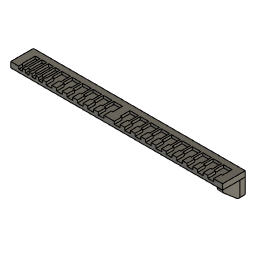
CClampRack v7 (Autodesk Fusion 360 design; units mm, degrees)
Autodesk Fusion 360 part; units mm, degrees
sketch "Sketch1" plane through (0, 0, 0) normal (0, 0, 1) x (1, 0, 0)
  line L0 (0, 76.2) -> (0, 0)
  line L1 (114.3, 57.15) -> (142.875, 57.15)
  line L2 (142.875, 57.15) -> (142.875, 25.4)
  line L3 (142.875, 25.4) -> (114.3, 25.4)
  line L4 (114.3, 25.4) -> (114.3, 57.15)
  line L5 (128.5875, 25.4) -> (128.5875, 0) construction
  line L6 (119.0625, 25.4) -> (119.0625, 0)
  line L7 (138.1125, 25.4) -> (138.1125, 0)
  line L8 (25.4, 57.15) -> (25.4, 12.7)
  line L9 (25.4, 12.7) -> (41.275, 12.7)
  line L10 (41.275, 12.7) -> (41.275, 57.15)
  line L11 (26.9875, 12.7) -> (26.9875, 0)
  line L12 (39.6875, 12.7) -> (39.6875, 0)
  line L13 (25.4, 57.15) -> (41.275, 57.15)
  line L14 (26.9875, 0) -> (39.6875, 0)
  line L15 (119.0625, 0) -> (138.1125, 0)
  line L16 (49.2125, 0) -> (61.9125, 0)
  line L17 (47.625, 57.15) -> (63.5, 57.15)
  line L18 (61.9125, 12.7) -> (61.9125, 0)
  line L19 (47.625, 57.15) -> (47.625, 12.7)
  line L20 (49.2125, 12.7) -> (49.2125, 0)
  line L21 (47.625, 12.7) -> (63.5, 12.7)
  line L22 (63.5, 12.7) -> (63.5, 57.15)
  line L23 (71.4375, 0) -> (84.1375, 0)
  line L24 (69.85, 57.15) -> (85.725, 57.15)
  line L25 (84.1375, 12.7) -> (84.1375, 0)
  line L26 (69.85, 57.15) -> (69.85, 12.7)
  line L27 (71.4375, 12.7) -> (71.4375, 0)
  line L28 (69.85, 12.7) -> (85.725, 12.7)
  line L29 (85.725, 12.7) -> (85.725, 57.15)
  line L30 (93.6625, 0) -> (106.3625, 0)
  line L31 (92.075, 57.15) -> (107.95, 57.15)
  line L32 (106.3625, 12.7) -> (106.3625, 0)
  line L33 (92.075, 57.15) -> (92.075, 12.7)
  line L34 (93.6625, 12.7) -> (93.6625, 0)
  line L35 (92.075, 12.7) -> (107.95, 12.7)
  line L36 (107.95, 12.7) -> (107.95, 57.15)
  line L37 (153.9875, 25.4) -> (153.9875, 0)
  line L38 (149.225, 57.15) -> (177.8, 57.15)
  line L39 (163.5125, 25.4) -> (163.5125, 0) construction
  line L40 (149.225, 25.4) -> (149.225, 57.15)
  line L41 (177.8, 25.4) -> (149.225, 25.4)
  line L42 (177.8, 57.15) -> (177.8, 25.4)
  line L43 (173.0375, 25.4) -> (173.0375, 0)
  line L44 (153.9875, 0) -> (173.0375, 0)
  line L45 (188.9125, 25.4) -> (188.9125, 0)
  line L46 (184.15, 57.15) -> (212.725, 57.15)
  line L47 (198.4375, 25.4) -> (198.4375, 0) construction
  line L48 (184.15, 25.4) -> (184.15, 57.15)
  line L49 (212.725, 25.4) -> (184.15, 25.4)
  line L50 (212.725, 57.15) -> (212.725, 25.4)
  line L51 (207.9625, 25.4) -> (207.9625, 0)
  line L52 (188.9125, 0) -> (207.9625, 0)
  line L53 (223.8375, 25.4) -> (223.8375, 0)
  line L54 (219.075, 57.15) -> (247.65, 57.15)
  line L55 (233.3625, 25.4) -> (233.3625, 0) construction
  line L56 (219.075, 25.4) -> (219.075, 57.15)
  line L57 (247.65, 25.4) -> (219.075, 25.4)
  line L58 (247.65, 57.15) -> (247.65, 25.4)
  line L59 (242.8875, 25.4) -> (242.8875, 0)
  line L60 (223.8375, 0) -> (242.8875, 0)
  line L61 (711.2, 76.2) -> (711.2, 0)
  line L62 (711.2, 0) -> (0, 0)
  line L63 (711.2, 76.2) -> (0, 76.2)
  line L64 (277.8125, 25.4) -> (277.8125, 0)
  line L65 (254, 57.15) -> (282.575, 57.15)
  line L66 (268.2875, 25.4) -> (268.2875, 0) construction
  line L67 (258.7625, 25.4) -> (258.7625, 0)
  line L68 (282.575, 25.4) -> (254, 25.4)
  line L69 (258.7625, 0) -> (277.8125, 0)
  line L70 (282.575, 57.15) -> (282.575, 25.4)
  line L71 (254, 25.4) -> (254, 57.15)
  line L72 (312.7375, 25.4) -> (312.7375, 0)
  line L73 (288.925, 57.15) -> (317.5, 57.15)
  line L74 (303.2125, 25.4) -> (303.2125, 0) construction
  line L75 (293.6875, 25.4) -> (293.6875, 0)
  line L76 (317.5, 25.4) -> (288.925, 25.4)
  line L77 (293.6875, 0) -> (312.7375, 0)
  line L78 (317.5, 57.15) -> (317.5, 25.4)
  line L79 (288.925, 25.4) -> (288.925, 57.15)
  line L80 (366.7125, 25.4) -> (366.7125, 0)
  line L81 (371.475, 25.4) -> (342.9, 25.4)
  line L82 (342.9, 57.15) -> (371.475, 57.15)
  line L83 (342.9, 25.4) -> (342.9, 57.15)
  line L84 (371.475, 57.15) -> (371.475, 25.4)
  line L85 (357.1875, 25.4) -> (357.1875, 0) construction
  line L86 (347.6625, 25.4) -> (347.6625, 0)
  line L87 (347.6625, 0) -> (366.7125, 0)
  line L88 (401.6375, 25.4) -> (401.6375, 0)
  line L89 (406.4, 25.4) -> (377.825, 25.4)
  line L90 (377.825, 57.15) -> (406.4, 57.15)
  line L91 (377.825, 25.4) -> (377.825, 57.15)
  line L92 (406.4, 57.15) -> (406.4, 25.4)
  line L93 (392.1125, 25.4) -> (392.1125, 0) construction
  line L94 (382.5875, 25.4) -> (382.5875, 0)
  line L95 (382.5875, 0) -> (401.6375, 0)
  line L96 (436.5625, 25.4) -> (436.5625, 0)
  line L97 (441.325, 25.4) -> (412.75, 25.4)
  line L98 (412.75, 57.15) -> (441.325, 57.15)
  line L99 (412.75, 25.4) -> (412.75, 57.15)
  line L100 (441.325, 57.15) -> (441.325, 25.4)
  line L101 (427.0375, 25.4) -> (427.0375, 0) construction
  line L102 (417.5125, 25.4) -> (417.5125, 0)
  line L103 (417.5125, 0) -> (436.5625, 0)
  line L104 (471.4875, 25.4) -> (471.4875, 0)
  line L105 (476.25, 25.4) -> (447.675, 25.4)
  line L106 (447.675, 57.15) -> (476.25, 57.15)
  line L107 (447.675, 25.4) -> (447.675, 57.15)
  line L108 (476.25, 57.15) -> (476.25, 25.4)
  line L109 (461.9625, 25.4) -> (461.9625, 0) construction
  line L110 (452.4375, 25.4) -> (452.4375, 0)
  line L111 (452.4375, 0) -> (471.4875, 0)
  line L112 (506.4125, 25.4) -> (506.4125, 0)
  line L113 (511.175, 25.4) -> (482.6, 25.4)
  line L114 (482.6, 57.15) -> (511.175, 57.15)
  line L115 (482.6, 25.4) -> (482.6, 57.15)
  line L116 (511.175, 57.15) -> (511.175, 25.4)
  line L117 (496.8875, 25.4) -> (496.8875, 0) construction
  line L118 (487.3625, 25.4) -> (487.3625, 0)
  line L119 (487.3625, 0) -> (506.4125, 0)
  line L120 (541.3375, 25.4) -> (541.3375, 0)
  line L121 (546.1, 25.4) -> (517.525, 25.4)
  line L122 (517.525, 57.15) -> (546.1, 57.15)
  line L123 (517.525, 25.4) -> (517.525, 57.15)
  line L124 (546.1, 57.15) -> (546.1, 25.4)
  line L125 (531.8125, 25.4) -> (531.8125, 0) construction
  line L126 (522.2875, 25.4) -> (522.2875, 0)
  line L127 (522.2875, 0) -> (541.3375, 0)
  line L128 (576.2625, 25.4) -> (576.2625, 0)
  line L129 (581.025, 25.4) -> (552.45, 25.4)
  line L130 (552.45, 57.15) -> (581.025, 57.15)
  line L131 (552.45, 25.4) -> (552.45, 57.15)
  line L132 (581.025, 57.15) -> (581.025, 25.4)
  line L133 (566.7375, 25.4) -> (566.7375, 0) construction
  line L134 (557.2125, 25.4) -> (557.2125, 0)
  line L135 (557.2125, 0) -> (576.2625, 0)
  line L136 (611.1875, 25.4) -> (611.1875, 0)
  line L137 (615.95, 25.4) -> (587.375, 25.4)
  line L138 (587.375, 57.15) -> (615.95, 57.15)
  line L139 (587.375, 25.4) -> (587.375, 57.15)
  line L140 (615.95, 57.15) -> (615.95, 25.4)
  line L141 (601.6625, 25.4) -> (601.6625, 0) construction
  line L142 (592.1375, 25.4) -> (592.1375, 0)
  line L143 (592.1375, 0) -> (611.1875, 0)
  line L144 (646.1125, 25.4) -> (646.1125, 0)
  line L145 (650.875, 25.4) -> (622.3, 25.4)
  line L146 (622.3, 57.15) -> (650.875, 57.15)
  line L147 (622.3, 25.4) -> (622.3, 57.15)
  line L148 (650.875, 57.15) -> (650.875, 25.4)
  line L149 (636.5875, 25.4) -> (636.5875, 0) construction
  line L150 (627.0625, 25.4) -> (627.0625, 0)
  line L151 (627.0625, 0) -> (646.1125, 0)
  line L152 (681.0375, 25.4) -> (681.0375, 0)
  line L153 (685.8, 25.4) -> (657.225, 25.4)
  line L154 (657.225, 57.15) -> (685.8, 57.15)
  line L155 (657.225, 25.4) -> (657.225, 57.15)
  line L156 (685.8, 57.15) -> (685.8, 25.4)
  line L157 (671.5125, 25.4) -> (671.5125, 0) construction
  line L158 (661.9875, 25.4) -> (661.9875, 0)
  line L159 (661.9875, 0) -> (681.0375, 0)
  dimension "d2" = 76.2
  dimension "d4" = 28.575
  dimension "d6" = 9.525
  dimension "d7" = 9.525
  dimension "d21" = 15.875
  dimension "d23" = 12.7
  dimension "d24" = 1.5875
  dimension "d25" = 15.875
  dimension "d26" = 12.7
  dimension "d27" = 1.5875
  dimension "d28" = 15.875
  dimension "d29" = 12.7
  dimension "d30" = 1.5875
  dimension "d31" = 15.875
  dimension "d32" = 12.7
  dimension "d33" = 1.5875
  dimension "d34" = 6.35
  dimension "d35" = 6.35
  dimension "d36" = 6.35
  dimension "d37" = 25.4
  dimension "d38" = 6.35
  dimension "d39" = 31.75
  dimension "d40" = 28.575
  dimension "d41" = 9.525
  dimension "d42" = 9.525
  dimension "d43" = 31.75
  dimension "d44" = 28.575
  dimension "d45" = 9.525
  dimension "d46" = 9.525
  dimension "d47" = 31.75
  dimension "d48" = 28.575
  dimension "d49" = 9.525
  dimension "d50" = 9.525
  dimension "d51" = 31.75
  dimension "d52" = 6.35
  dimension "d53" = 6.35
  dimension "d54" = 6.35
  dimension "d56" = 28.575
  dimension "d57" = 9.525
  dimension "d58" = 9.525
  dimension "d59" = 31.75
  dimension "d60" = 28.575
  dimension "d61" = 9.525
  dimension "d62" = 9.525
  dimension "d63" = 31.75
  dimension "d64" = 6.35
  dimension "d65" = 6.35
  dimension "d81" = 28.575
  dimension "d82" = 9.525
  dimension "d83" = 9.525
  dimension "d84" = 31.75
  dimension "d85" = 28.575
  dimension "d86" = 9.525
  dimension "d87" = 9.525
  dimension "d88" = 31.75
  dimension "d89" = 28.575
  dimension "d90" = 9.525
  dimension "d91" = 9.525
  dimension "d92" = 31.75
  dimension "d93" = 28.575
  dimension "d94" = 9.525
  dimension "d95" = 9.525
  dimension "d96" = 31.75
  dimension "d97" = 28.575
  dimension "d98" = 9.525
  dimension "d99" = 9.525
  dimension "d100" = 31.75
  dimension "d101" = 28.575
  dimension "d102" = 9.525
  dimension "d103" = 9.525
  dimension "d104" = 31.75
  dimension "d105" = 28.575
  dimension "d106" = 9.525
  dimension "d107" = 9.525
  dimension "d108" = 31.75
  dimension "d109" = 28.575
  dimension "d110" = 9.525
  dimension "d111" = 9.525
  dimension "d112" = 31.75
  dimension "d113" = 28.575
  dimension "d114" = 9.525
  dimension "d115" = 9.525
  dimension "d116" = 31.75
  dimension "d117" = 28.575
  dimension "d118" = 9.525
  dimension "d119" = 9.525
  dimension "d120" = 31.75
  dimension "d121" = 25.4
  dimension "d122" = 6.35
  dimension "d123" = 6.35
  dimension "d124" = 6.35
  dimension "d125" = 6.35
  dimension "d126" = 6.35
  dimension "d127" = 6.35
  dimension "d128" = 6.35
  dimension "d129" = 6.35
  dimension "d130" = 6.35
  dimension "d131" = 25.4
  constraint vertical L0
  constraint horizontal L1
  constraint horizontal L3
  constraint vertical L4
  constraint midpoint L3 L5.start
  constraint coincident L3 L6.start
  constraint coincident L3 L7.start
  constraint perpendicular L8 L9
  constraint coincident L9 L11.start
  constraint coincident L9 L12.start
  constraint perpendicular L10 L13
  constraint perpendicular L12 L14
  constraint perpendicular L7 L15
  constraint perpendicular L19 L21
  constraint coincident L20.start L21
  constraint coincident L18.start L21
  constraint perpendicular L17 L22
  constraint perpendicular L16 L18
  constraint perpendicular L26 L28
  constraint coincident L27.start L28
  constraint coincident L25.start L28
  constraint perpendicular L24 L29
  constraint perpendicular L23 L25
  constraint perpendicular L33 L35
  constraint coincident L34.start L35
  constraint coincident L32.start L35
  constraint perpendicular L31 L36
  constraint perpendicular L30 L32
  constraint perpendicular L2 L3
  constraint horizontal L38
  constraint horizontal L41
  constraint vertical L40
  constraint midpoint L39.start L41
  constraint coincident L37.start L41
  constraint coincident L43.start L41
  constraint perpendicular L43 L44
  constraint perpendicular L41 L42
  constraint horizontal L46
  constraint horizontal L49
  constraint vertical L48
  constraint midpoint L47.start L49
  constraint coincident L45.start L49
  constraint coincident L51.start L49
  constraint perpendicular L51 L52
  constraint perpendicular L49 L50
  constraint horizontal L54
  constraint horizontal L57
  constraint vertical L56
  constraint midpoint L55.start L57
  constraint coincident L53.start L57
  constraint coincident L59.start L57
  constraint perpendicular L59 L60
  constraint perpendicular L57 L58
  constraint coincident L0.end L62.end
  constraint collinear L1 L31
  constraint perpendicular L54 L61
  constraint perpendicular L0 L62
  constraint equal L0 L61
  constraint horizontal L65
  constraint horizontal L68
  constraint vertical L71
  constraint midpoint L66.start L68
  constraint coincident L67.start L68
  constraint coincident L64.start L68
  constraint perpendicular L64 L69
  constraint perpendicular L68 L70
  constraint horizontal L73
  constraint horizontal L76
  constraint vertical L79
  constraint midpoint L74.start L76
  constraint coincident L75.start L76
  constraint coincident L72.start L76
  constraint perpendicular L72 L77
  constraint perpendicular L76 L78
  constraint horizontal L82
  constraint horizontal L81
  constraint vertical L83
  constraint midpoint L85.start L81
  constraint coincident L86.start L81
  constraint coincident L80.start L81
  constraint perpendicular L80 L87
  constraint perpendicular L81 L84
  constraint horizontal L90
  constraint horizontal L89
  constraint vertical L91
  constraint midpoint L93.start L89
  constraint coincident L94.start L89
  constraint coincident L88.start L89
  constraint perpendicular L88 L95
  constraint perpendicular L89 L92
  constraint horizontal L98
  constraint horizontal L97
  constraint vertical L99
  constraint midpoint L101.start L97
  constraint coincident L102.start L97
  constraint coincident L96.start L97
  constraint perpendicular L96 L103
  constraint perpendicular L97 L100
  constraint horizontal L106
  constraint horizontal L105
  constraint vertical L107
  constraint midpoint L109.start L105
  constraint coincident L110.start L105
  constraint coincident L104.start L105
  constraint perpendicular L104 L111
  constraint perpendicular L105 L108
  constraint horizontal L114
  constraint horizontal L113
  constraint vertical L115
  constraint midpoint L117.start L113
  constraint coincident L118.start L113
  constraint coincident L112.start L113
  constraint perpendicular L112 L119
  constraint perpendicular L113 L116
  constraint horizontal L122
  constraint horizontal L121
  constraint vertical L123
  constraint midpoint L125.start L121
  constraint coincident L126.start L121
  constraint coincident L120.start L121
  constraint perpendicular L120 L127
  constraint perpendicular L121 L124
  constraint horizontal L130
  constraint horizontal L129
  constraint vertical L131
  constraint midpoint L133.start L129
  constraint coincident L134.start L129
  constraint coincident L128.start L129
  constraint perpendicular L128 L135
  constraint perpendicular L129 L132
  constraint horizontal L138
  constraint horizontal L137
  constraint vertical L139
  constraint midpoint L141.start L137
  constraint coincident L142.start L137
  constraint coincident L136.start L137
  constraint perpendicular L136 L143
  constraint perpendicular L137 L140
  constraint horizontal L146
  constraint horizontal L145
  constraint vertical L147
  constraint midpoint L149.start L145
  constraint coincident L150.start L145
  constraint coincident L144.start L145
  constraint perpendicular L144 L151
  constraint perpendicular L145 L148
  constraint horizontal L154
  constraint horizontal L153
  constraint vertical L155
  constraint midpoint L157.start L153
  constraint coincident L158.start L153
  constraint coincident L152.start L153
  constraint perpendicular L152 L159
  constraint perpendicular L153 L156
  measures "d2" distance of L0.end L0.start
  measures "d4" horizontal distance of L1.start L1.end
  measures "d6" distance of L5 L6
  measures "d7" distance of L5 L7
  measures "d21" distance of L8 L10
  measures "d23" distance of L11 L12
  measures "d24" distance of L8 L11
  measures "d25" distance of L19 L22
  measures "d26" distance of L18 L20
  measures "d27" distance of L19 L20
  measures "d28" distance of L26 L29
  measures "d29" distance of L25 L27
  measures "d30" distance of L26 L27
  measures "d31" distance of L33 L36
  measures "d32" distance of L32 L34
  measures "d33" distance of L33 L34
  measures "d34" distance of L10 L19
  measures "d35" distance of L22 L26
  measures "d36" distance of L29 L33
  measures "d37" distance of L0 L8
  measures "d38" distance of L4 L36
  measures "d39" vertical distance of L1.end L2.end
  measures "d40" horizontal distance of L38.start L38.end
  measures "d41" distance of L37 L39
  measures "d42" distance of L39 L43
  measures "d43" vertical distance of L38.end L41.start
  measures "d44" horizontal distance of L46.start L46.end
  measures "d45" distance of L45 L47
  measures "d46" distance of L47 L51
  measures "d47" vertical distance of L46.end L49.start
  measures "d48" horizontal distance of L54.start L54.end
  measures "d49" distance of L53 L55
  measures "d50" distance of L55 L59
  measures "d51" vertical distance of L54.end L57.start
  measures "d52" distance of L2 L40
  measures "d53" distance of L42 L48
  measures "d54" distance of L50 L56
  measures "d56" horizontal distance of L65.start L65.end
  measures "d57" distance of L66 L67
  measures "d58" distance of L64 L66
  measures "d59" vertical distance of L65.end L68.start
  measures "d60" horizontal distance of L73.start L73.end
  measures "d61" distance of L74 L75
  measures "d62" distance of L72 L74
  measures "d63" vertical distance of L73.end L76.start
  measures "d64" distance of L58 L71
  measures "d65" distance of L70 L79
  measures "d81" horizontal distance of L82.start L82.end
  measures "d82" distance of L85 L86
  measures "d83" distance of L80 L85
  measures "d84" vertical distance of L82.end L81.start
  measures "d85" horizontal distance of L90.start L90.end
  measures "d86" distance of L93 L94
  measures "d87" distance of L88 L93
  measures "d88" vertical distance of L90.end L89.start
  measures "d89" horizontal distance of L98.start L98.end
  measures "d90" distance of L101 L102
  measures "d91" distance of L96 L101
  measures "d92" vertical distance of L98.end L97.start
  measures "d93" horizontal distance of L106.start L106.end
  measures "d94" distance of L109 L110
  measures "d95" distance of L104 L109
  measures "d96" vertical distance of L106.end L105.start
  measures "d97" horizontal distance of L114.start L114.end
  measures "d98" distance of L117 L118
  measures "d99" distance of L112 L117
  measures "d100" vertical distance of L114.end L113.start
  measures "d101" horizontal distance of L122.start L122.end
  measures "d102" distance of L125 L126
  measures "d103" distance of L120 L125
  measures "d104" vertical distance of L122.end L121.start
  measures "d105" horizontal distance of L130.start L130.end
  measures "d106" distance of L133 L134
  measures "d107" distance of L128 L133
  measures "d108" vertical distance of L130.end L129.start
  measures "d109" horizontal distance of L138.start L138.end
  measures "d110" distance of L141 L142
  measures "d111" distance of L136 L141
  measures "d112" vertical distance of L138.end L137.start
  measures "d113" horizontal distance of L146.start L146.end
  measures "d114" distance of L149 L150
  measures "d115" distance of L144 L149
  measures "d116" vertical distance of L146.end L145.start
  measures "d117" horizontal distance of L154.start L154.end
  measures "d118" distance of L157 L158
  measures "d119" distance of L152 L157
  measures "d120" vertical distance of L154.end L153.start
  measures "d121" distance of L78 L83
  measures "d122" distance of L84 L91
  measures "d123" distance of L92 L99
  measures "d124" distance of L100 L107
  measures "d125" distance of L108 L115
  measures "d126" distance of L116 L123
  measures "d127" distance of L124 L131
  measures "d128" distance of L132 L139
  measures "d129" distance of L140 L147
  measures "d130" distance of L148 L155
  measures "d131" distance of L61 L156
extrude "Extrude10" add sketch "Sketch1" against normal blind 18.2563 makes body 1
extrude "Extrude11" cut sketch "Sketch1" against normal blind 8.89 contours L9 L11 L12 L14 L62 | L8 L9 L10 L13 | L62 L152 L153 L158 L159 | L16 L18 L20 L21 L62 | L153 L154 L155 L156 | L17 L19 L21 L22 | L62 L144 L145 L150 L151 | L23 L25 L27 L28 L62 | L145 L146 L147 L148 | L24 L26 L28 L29 | L62 L136 L137 L142 L143 | L30 L32 L34 L35 L62 | L137 L138 L139 L140 | L31 L33 L35 L36 | L62 L128 L129 L134 L135 | L3 L6 L7 L15 L62 | L129 L130 L131 L132 | L1 L2 L3 L4 | L62 L120 L121 L126 L127 | L37 L41 L43 L44 L62 | L121 L122 L123 L124 | L38 L40 L41 L42 | L62 L112 L113 L118 L119 | L45 L49 L51 L52 L62 | L113 L114 L115 L116 | L46 L48 L49 L50 | L62 L104 L105 L110 L111 | L53 L57 L59 L60 L62 | L105 L106 L107 L108 | L54 L56 L57 L58 | L62 L96 L97 L102 L103 | L62 L64 L67 L68 L69 | L97 L98 L99 L100 | L65 L68 L70 L71 | L62 L88 L89 L94 L95 | L62 L72 L75 L76 L77 | L89 L90 L91 L92 | L73 L76 L78 L79 | L62 L80 L81 L86 L87 | L81 L82 L83 L84 bodies 1
sketch "Sketch4" plane through (0, 0, -18.2563) normal (0, 0, -1) x (1, 0, 0)
  line L0 (711.2, 0) -> (0, 0)
  line L1 (0, 0) -> (0, -76.2)
  line L2 (0, -76.2) -> (711.2, -76.2)
  line L3 (711.2, -76.2) -> (711.2, 0)
  line L4 (0, -76.2) -> (711.2, -76.2)
  line L5 (711.2, -76.2) -> (711.2, -57.9438)
  line L6 (711.2, -57.9438) -> (0, -57.9438)
  line L7 (0, -57.9438) -> (0, -76.2)
  dimension "d136" = 18.2563
  constraint horizontal L4
  constraint vertical L5
  constraint horizontal L6
  constraint vertical L7
  constraint coincident L1.end L2.start
  measures "d136" distance of L1.end L6.end
extrude "Extrude12" add sketch "Sketch4" along normal blind 50.8 separate body contours L1 L2 L3 L4 L5 L6 L7 makes body 2
sketch "Sketch5" plane through (711.2, 0, 0) normal (1, 0, 0) x (0, 1, 0)
  line L0 (76.2, 0) -> (0, 0)
  line L1 (0, 0) -> (0, -18.2563)
  line L2 (0, -18.2563) -> (76.2, -18.2563)
  line L3 (76.2, -18.2563) -> (76.2, 0)
  line L4 (76.2, 0) -> (0, 0)
  line L5 (76.2, 0) -> (76.2, -18.2563)
  line L6 (76.2, -18.2563) -> (76.2, -69.0563)
  line L7 (76.2, -69.0563) -> (57.9438, -69.0563)
  line L8 (0, 0) -> (0, -19.5687)
  line L9 (4.4226, -29.2006) -> (47.2299, -65.9882)
  line L10 (55.5073, -69.0563) -> (57.9438, -69.0563)
  arc A0 (0, -19.5687) -> (4.4226, -29.2006) centre (12.7, -19.5687) ccw
  arc A1 (47.2299, -65.9882) -> (55.5073, -69.0563) centre (55.5073, -56.3562) ccw
  line L11 (57.9438, -69.0563) -> (57.9438, -18.2563)
  line L12 (57.9438, -18.2563) -> (0, -18.2563)
  point P0 (0, -25.4)
  point P1 (50.8, -69.0562)
  dimension "d139" = 25.4
  dimension "d140" = 25.4
  dimension "d141" = 12.7
  dimension "d142" = 12.7
  constraint coincident L0.end L1.start
  constraint perpendicular L0 L8
  constraint coincident L7.end L10.end
  constraint perpendicular L1 L10
  constraint coincident P0 L8
  constraint coincident P0 L9
  constraint tangent L8 A0
  constraint tangent L9 A0
  constraint coincident P1 L9
  constraint coincident P1 L10
  constraint tangent L9 A1
  constraint tangent L10 A1
  constraint coincident L2 L11.end
  constraint perpendicular L2 L11
  constraint coincident L1.end L2.start
  measures "d139" distance of L0.end P0
  measures "d140" distance of L6.end P1
  measures "d141" radius of A0
  measures "d142" radius of A1
extrude "Extrude13" add sketch "Sketch5" against normal blind 18.2563 separate body contours L2 L8 L9 L10 A0 A1 L11 L12 makes body 3
equation "d21 = ( 5 / 8 ) * 1 in"
equation "d24 = ( 1 / 16 ) * 1 in"
equation "d25 = ( 5 / 8 ) * 1 in"
equation "d27 = ( 1 / 16 ) * 1 in"
equation "d28 = ( 5 / 8 ) * 1 in"
equation "d30 = ( 1 / 16 ) * 1 in"
equation "d31 = ( 5 / 8 ) * 1 in"
equation "d33 = ( 1 / 16 ) * 1 in"
equation "d132 = ( -23 / 32 ) * 1 in"
equation "d136 = ( 23 / 32 ) * 1 in"
equation "d143 = ( -23 / 32 ) * 1 in"
